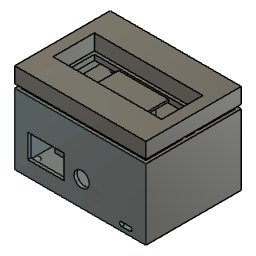
Todas la partes de la carcasa v1 (Autodesk Fusion 360 design; units mm, degrees)
Autodesk Fusion 360 part; units mm, degrees
(part 1 of 4)
sketch "Boceto1" plane through (0, 0, 0) normal (0, 1, 0) x (1, 0, 0)
sketch "Boceto2" plane through (0, 0, 0) normal (0, 1, 0) x (1, 0, 0)
  line L0 (-80, 70) -> (41, 70)
  line L1 (41, 70) -> (41, -16.3)
  line L2 (41, -16.3) -> (-80, -16.3)
  line L3 (-80, -16.3) -> (-80, 70)
  line L4 (44, -19.3) -> (-83, -19.3)
  line L5 (-83, -19.3) -> (-83, 73)
  line L6 (-83, 73) -> (44, 73)
  line L7 (44, 73) -> (44, -19.3)
  dimension "d1" = 121
  dimension "d2" = 86.3
  dimension "d3" = -3
  constraint horizontal L0
  constraint vertical L1
  constraint horizontal L2
  constraint vertical L3
  measures "d1" distance of L0.start L0.end
  measures "d2" distance of L0.end L1.end
extrude "Extruir1" add sketch "Boceto2" along normal blind 64.2 makes body 1
sketch "Boceto3" plane through (0, 0, 0) normal (0, 1, 0) x (1, 0, 0)
  line L0 (41, 70) -> (41, -16.3)
  line L1 (44, -19.3) -> (44, 73)
extrude "Extruir3" add sketch "Boceto2" against normal blind 4 contours L0 L1 L2 L3 | L4 L5 L6 L7 bodies 1
sketch "Boceto4" plane through (0, 0, 0) normal (0, 1, 0) x (1, 0, 0)
  line L0 (-47.2876, 12.1063) -> (-72.5876, 12.1063)
  line L1 (-45.7876, 61.8063) -> (-45.7876, 13.6063)
  circle A0 centre (-48.1876, 61.0063) radius 1.45
  circle A1 centre (-48.1876, 14.4063) radius 1.45
  line L2 (-72.5876, 12.1063) -> (-74.0876, 13.6063)
  line L3 (-47.2876, 12.1063) -> (-45.7876, 13.6063)
  circle A2 centre (-71.6876, 14.4063) radius 1.45
  line L4 (-45.7876, 13.6063) -> (-45.7876, 61.8063)
  line L5 (-45.7876, 61.8063) -> (-47.2876, 63.3063)
  circle A3 centre (-71.6876, 14.4063) radius 1.45
  line L6 (-72.5876, 63.3063) -> (-47.2876, 63.3063)
  line L7 (-74.0876, 13.6063) -> (-72.5876, 12.1063)
  line L8 (-74.0876, 61.8063) -> (-72.5876, 63.3063)
  circle A4 centre (-71.6876, 61.0063) radius 1.45
  line L9 (-72.5876, 12.1063) -> (-47.2876, 12.1063)
  line L10 (-72.5876, 63.3063) -> (-74.0876, 61.8063)
  line L11 (-74.0876, 61.8063) -> (-74.0876, 13.6063)
  circle A5 centre (-71.6876, 61.0063) radius 1.45
  line L12 (-74.0876, 13.6063) -> (-74.0876, 61.8063)
  circle A6 centre (-48.1876, 61.0063) radius 1.45
  line L13 (-47.2876, 63.3063) -> (-72.5876, 63.3063)
  line L14 (-45.7876, 13.6063) -> (-47.2876, 12.1063)
  line L15 (-47.2876, 63.3063) -> (-45.7876, 61.8063)
  circle A7 centre (-48.1876, 14.4063) radius 1.45
  line L16 (-43.7876, 12.7779) -> (-46.4591, 10.1063)
  line L17 (-73.416, 10.1063) -> (-46.4591, 10.1063)
  line L18 (-73.416, 10.1063) -> (-76.0876, 12.7779)
  line L19 (-76.0876, 62.6347) -> (-76.0876, 12.7779)
  line L20 (-76.0876, 62.6347) -> (-73.416, 65.3063)
  line L21 (-46.4591, 65.3063) -> (-73.416, 65.3063)
  line L22 (-46.4591, 65.3063) -> (-43.7876, 62.6347)
  line L23 (-43.7876, 62.6347) -> (-43.7876, 12.7779)
  point P0 (-45.7876, 63.3063)
  dimension "d10" = -2
sketch "Boceto5" plane through (0, 0, 0) normal (0, 1, 0) x (1, 0, 0)
extrude "Extruir4" add sketch "Boceto4" along normal blind 11 contours L16 L17 L18 L19 L20 L21 L22 L23 bodies 1
extrude "Extruir5" add sketch "Boceto4" along normal blind 9.866 contours A0 A6 | A1 A7 | A2 A3 | A4 A5 bodies 1
sketch "Boceto6" plane through (0, 0, 19.3) normal (0, 0, 1) x (1, 0, 0)
  line L0 (-70.6711, 11.1811) -> (-35.0211, 11.1811)
  line L1 (-35.0211, 34.2811) -> (-46.6399, 34.2811)
  circle A0 centre (-37.6711, 8.3311) radius 1.45
  line L2 (-35.0211, 39.3811) -> (-35.0211, 30.3811)
  line L3 (-45.8461, 39.3811) -> (-35.0211, 39.3811)
  line L4 (-70.6711, 34.2811) -> (-70.6711, 11.1811)
  line L5 (-35.0211, 5.7811) -> (-70.6711, 5.7811)
  line L6 (-35.0211, 11.1811) -> (-35.0211, 34.2811)
  line L7 (-59.0499, 34.2811) -> (-70.6711, 34.2811)
  line L8 (-46.6399, 34.2811) -> (-59.0499, 34.2811)
  circle A1 centre (-37.6711, 36.9311) radius 1.45
  line L9 (-35.0211, 11.1811) -> (-35.0211, 5.7811)
  circle A2 centre (-37.6711, 36.8311) radius 1.45
  line L10 (-35.0211, 33.9811) -> (-35.0211, 10.8811)
  line L11 (-45.8461, 5.7811) -> (-45.8461, 9.5311)
  line L12 (-59.8461, 9.5311) -> (-59.8461, 5.7811)
  line L13 (-70.6711, 14.7811) -> (-70.6711, 5.7811)
  line L14 (-46.6399, 10.8811) -> (-59.0499, 10.8811)
  line L15 (-35.0211, 33.9811) -> (-35.0211, 39.3811)
  line L16 (-70.6711, 10.8811) -> (-70.6711, 33.9811)
  line L17 (-59.0499, 10.8811) -> (-70.6711, 10.8811)
  line L18 (-45.8461, 9.5311) -> (-59.8461, 9.5311)
  line L19 (-70.6711, 5.7811) -> (-59.8461, 5.7811)
  line L20 (-35.0211, 39.3811) -> (-70.6711, 39.3811)
  line L21 (-70.6711, 39.3811) -> (-70.6711, 33.9811)
  line L22 (-70.6711, 33.9811) -> (-35.0211, 33.9811)
  line L23 (-35.0211, 10.8811) -> (-46.6399, 10.8811)
  line L24 (-35.0211, 5.7811) -> (-35.0211, 14.7811)
  circle A3 centre (-37.6711, 8.2311) radius 1.45
  circle A4 centre (-68.0211, 8.2311) radius 1.45
  circle A5 centre (-68.0211, 36.8311) radius 1.45
  point P0 (-52.8461, 22.5811)
  point P1 (-52.8461, 22.5811)
sketch "Boceto7" plane through (0, 0, 0) normal (0, 1, 0) x (1, 0, 0)
  line L0 (-6.4734, 52.2282) -> (33.9266, 52.2282)
  line L1 (-6.4738, 51.7714) -> (-6.4738, 57.7714)
  arc A0 (33.9266, 52.2282) -> (33.9266, 57.2282) centre (33.9266, 54.7282) ccw
  line L2 (-16.6738, 51.7714) -> (-6.4738, 51.7714)
  line L3 (-16.6738, 57.7714) -> (-16.6738, 51.7714)
  line L4 (33.9266, 57.2282) -> (-6.4734, 57.2282)
  line L5 (-6.4738, 57.7714) -> (-16.6738, 57.7714)
  point P0 (11.2266, 57.2282)
sketch "Boceto8" plane through (0, 0, 0) normal (0, 1, 0) x (1, 0, 0)
  line L0 (-6.2702, 42.1492) -> (34.1298, 42.1492)
  line L1 (-6.2705, 41.6923) -> (-6.2705, 47.6923)
  arc A0 (34.1298, 42.1492) -> (34.1298, 47.1492) centre (34.1298, 44.6492) ccw
  line L2 (-16.4705, 41.6923) -> (-6.2705, 41.6923)
  line L3 (-16.4705, 47.6923) -> (-16.4705, 41.6923)
  line L4 (34.1298, 47.1492) -> (-6.2702, 47.1492)
  line L5 (-6.2705, 47.6923) -> (-16.4705, 47.6923)
  point P0 (11.4298, 47.1492)
sketch "Boceto9" plane through (0, 0, 0) normal (0, 1, 0) x (1, 0, 0)
  line L0 (-6.3461, 32.1874) -> (34.0539, 32.1874)
  line L1 (-6.3465, 31.7305) -> (-6.3465, 37.7305)
  arc A0 (34.0539, 32.1874) -> (34.0539, 37.1874) centre (34.0539, 34.6874) ccw
  line L2 (-16.5465, 31.7305) -> (-6.3465, 31.7305)
  line L3 (-16.5465, 37.7305) -> (-16.5465, 31.7305)
  line L4 (34.0539, 37.1874) -> (-6.3461, 37.1874)
  line L5 (-6.3465, 37.7305) -> (-16.5465, 37.7305)
  point P0 (11.3539, 37.1874)
sketch "Boceto10" plane through (0, 0, 0) normal (0, 1, 0) x (-1, 0, 0)
  line L0 (-41, 16.3) -> (-41, -70)
  line L1 (-41, -70) -> (80, -70)
  line L2 (80, -70) -> (80, 16.3)
  line L3 (80, 16.3) -> (-41, 16.3)
  line L4 (46.4591, -65.3063) -> (43.7876, -62.6347)
  line L5 (43.7876, -62.6347) -> (43.7876, -12.7779)
  line L6 (43.7876, -12.7779) -> (46.4591, -10.1063)
  line L7 (46.4591, -10.1063) -> (73.416, -10.1063)
  line L8 (73.416, -10.1063) -> (76.0876, -12.7779)
  line L9 (76.0876, -12.7779) -> (76.0876, -62.6347)
  line L10 (76.0876, -62.6347) -> (73.416, -65.3063)
  line L11 (73.416, -65.3063) -> (46.4591, -65.3063)
  line L12 (6.3465, -31.7305) -> (6.3465, -37.7305)
  line L13 (16.5465, -31.7305) -> (6.3465, -31.7305)
  line L14 (6.3465, -37.7305) -> (16.5465, -37.7305)
  line L15 (16.5465, -37.7305) -> (16.5465, -31.7305)
  line L16 (-34.0539, -37.1874) -> (6.3461, -37.1874)
  line L17 (6.3461, -32.1874) -> (-34.0539, -32.1874)
  arc A0 (-34.0539, -32.1874) -> (-34.0539, -37.1874) centre (-34.0539, -34.6874) ccw
  line L18 (6.2702, -42.1492) -> (-34.1298, -42.1492)
  arc A1 (-34.1298, -42.1492) -> (-34.1298, -47.1492) centre (-34.1298, -44.6492) ccw
  line L19 (-34.1298, -47.1492) -> (6.2702, -47.1492)
  line L20 (16.4705, -47.6923) -> (16.4705, -41.6923)
  line L21 (16.4705, -41.6923) -> (6.2705, -41.6923)
  line L22 (6.2705, -41.6923) -> (6.2705, -47.6923)
  line L23 (6.2705, -47.6923) -> (16.4705, -47.6923)
  line L24 (6.4734, -52.2282) -> (-33.9266, -52.2282)
  arc A2 (-33.9266, -52.2282) -> (-33.9266, -57.2282) centre (-33.9266, -54.7282) ccw
  line L25 (-33.9266, -57.2282) -> (6.4734, -57.2282)
  line L26 (6.4738, -57.7714) -> (16.6738, -57.7714)
  line L27 (6.4738, -51.7714) -> (6.4738, -57.7714)
  line L28 (16.6738, -57.7714) -> (16.6738, -51.7714)
  line L29 (16.6738, -51.7714) -> (6.4738, -51.7714)
  line L30 (-38.4075, -28.7305) -> (19.6738, -28.7305)
  line L31 (19.6738, -28.7305) -> (19.6738, -60.7714)
  line L32 (19.6738, -60.7714) -> (-38.4075, -60.7714)
  line L33 (-38.4075, -60.7714) -> (-38.4075, -28.7305)
  line L34 (16.6738, -57.7714) -> (19.6738, -57.7714) construction
  line L35 (16.6738, -57.7714) -> (16.6738, -60.7714) construction
  line L36 (16.5465, -31.7305) -> (16.5091, -28.7305) construction
  line L37 (-36.6075, -44.9828) -> (-38.4075, -44.9828) construction
  dimension "d19" = 3
  dimension "d20" = 3
  dimension "d21" = 3
  dimension "d22" = 1.8
  constraint horizontal L30
  constraint vertical L31
  constraint horizontal L32
  constraint vertical L33
  constraint coincident L26.end L28.start
  constraint coincident L31 L34.end
  constraint perpendicular L31 L34
  constraint coincident L32 L35.end
  constraint perpendicular L32 L35
  constraint coincident L13.start L15.end
  constraint coincident L30 L36.end
  constraint coincident A1 L37.start
  constraint coincident L33 L37.end
  constraint perpendicular L33 L37
  measures "d19" distance of L26.end L34.end
  measures "d20" distance of L26.end L35.end
  measures "d21" vertical distance of L13.start L36.end
  measures "d22" distance of L37.start L37.end
extrude "Extruir8" add sketch "Boceto10" along normal blind 15 contours L12 L16 L17 A0 | L18 A1 L19 L22 | L24 A2 L25 L27 | L30 L31 L32 L33 bodies 1
sketch "Boceto11" plane through (0, 0, 0) normal (0, 1, 0) x (1, 0, 0)
sketch "Boceto12" plane through (0, 15, 0) normal (0, 1, 0) x (-1, 0, 0)
  line L0 (6.4738, -51.7714) -> (16.6738, -51.7714)
  line L1 (16.6738, -51.7714) -> (16.6738, -57.7714)
  line L2 (16.6738, -57.7714) -> (6.4738, -57.7714)
  line L3 (6.4738, -57.7714) -> (6.4738, -51.7714)
  line L4 (16.5465, -31.7305) -> (16.5465, -37.7305)
  line L5 (16.5465, -37.7305) -> (6.3465, -37.7305)
  line L6 (6.3465, -37.7305) -> (6.3465, -31.7305)
  line L7 (6.3465, -31.7305) -> (16.5465, -31.7305)
  line L8 (16.4705, -47.6923) -> (6.2705, -47.6923)
  line L9 (6.2705, -47.6923) -> (6.2705, -41.6923)
  line L10 (6.2705, -41.6923) -> (16.4705, -41.6923)
  line L11 (16.4705, -41.6923) -> (16.4705, -47.6923)
  line L12 (-38.4075, -60.7714) -> (19.6738, -60.7714)
  line L13 (19.6738, -60.7714) -> (19.6738, -28.7305)
  line L14 (19.6738, -28.7305) -> (-38.4075, -28.7305)
  line L15 (-38.4075, -28.7305) -> (-38.4075, -60.7714)
  line L16 (-33.9266, -57.2282) -> (6.4734, -57.2282)
  arc A0 (-33.9266, -52.2282) -> (-33.9266, -57.2282) centre (-33.9266, -54.7282) ccw
  line L17 (6.4734, -52.2282) -> (-33.9266, -52.2282)
  line L18 (6.4734, -57.2282) -> (-33.9266, -57.2282)
  line L19 (-33.9266, -57.2282) -> (-33.9266, -52.2282)
  line L20 (-33.9266, -52.2282) -> (6.4734, -52.2282)
  line L21 (6.4734, -52.2282) -> (6.4734, -57.2282)
  line L22 (-34.1298, -47.1492) -> (6.2702, -47.1492)
  line L23 (6.2702, -42.1492) -> (-34.1298, -42.1492)
  arc A1 (-34.1298, -42.1492) -> (-34.1298, -47.1492) centre (-34.1298, -44.6492) ccw
  line L24 (-34.0539, -37.1874) -> (6.3461, -37.1874)
  line L25 (6.3461, -32.1874) -> (-34.0539, -32.1874)
  arc A2 (-34.0539, -32.1874) -> (-34.0539, -37.1874) centre (-34.0539, -34.6874) ccw
  line L26 (6.2702, -47.1492) -> (-34.1298, -47.1492)
  line L27 (-34.1298, -47.1492) -> (-34.1298, -42.1492)
  line L28 (-34.1298, -42.1492) -> (6.2702, -42.1492)
  line L29 (6.2702, -42.1492) -> (6.2702, -47.1492)
  line L30 (6.3461, -37.1874) -> (-34.0539, -37.1874)
  line L31 (-34.0539, -37.1874) -> (-34.0539, -32.1874)
  line L32 (-34.0539, -32.1874) -> (6.3461, -32.1874)
  line L33 (6.3461, -32.1874) -> (6.3461, -37.1874)
  constraint horizontal L18
  constraint vertical L19
  constraint horizontal L20
  constraint vertical L21
  constraint coincident A0.start L17.end
  constraint coincident L16.end L18.start
  constraint horizontal L26
  constraint vertical L27
  constraint horizontal L28
  constraint vertical L29
  constraint coincident L23.end A1.start
  constraint coincident L22.end L26.start
  constraint horizontal L30
  constraint vertical L31
  constraint horizontal L32
  constraint vertical L33
  constraint coincident L25.end A2.start
  constraint coincident L24.end L30.start
extrude "Extruir9" cut sketch "Boceto12" against normal blind 15 contours L16 L17 L18 L19 L20 L21 | A0 L19 | L22 L23 L26 L27 L28 L29 | A1 L27 | L24 L25 L30 L31 L32 L33 | A2 L31 bodies 1
extrude "Extruir10" cut 1 faces at (-6.3461, 10, -33.854) along direction (-1, 0, 0) blind 3 on bodies 1 bodies 1
extrude "Extruir11" cut 1 faces at (-6.2702, 10, -43.8159) along direction (-1, 0, 0) blind 3 on bodies 1 bodies 1
extrude "Extruir12" cut 1 faces at (-6.4734, 10, -53.8949) along direction (-1, 0, 0) blind 2 on bodies 1 bodies 1
sketch "Boceto13" plane through (0, 0, 19.3) normal (0, 0, 1) x (1, 0, 0)
  circle A0 centre (-23.7062, 31.534) radius 1.5
  line L0 (-10.9162, 11.184) -> (-13.4262, 11.184)
  line L1 (-26.2062, 35.884) -> (-7.2062, 35.884)
  line L2 (-7.2062, 13.634) -> (-26.2062, 13.634)
  line L3 (-23.7062, 9.634) -> (-23.7062, 35.884)
  line L4 (-8.4062, 35.884) -> (-8.4062, 9.634)
  line L5 (-18.4462, 11.184) -> (-20.9562, 11.184)
  line L6 (-18.4462, 13.634) -> (-15.9362, 13.634)
  line L7 (-15.9362, 11.184) -> (-15.9362, 13.634)
  line L8 (-7.2062, 9.634) -> (-26.2062, 9.634)
  circle A1 centre (-23.7062, 14.684) radius 1.5
  line L9 (-20.9562, 35.884) -> (-20.9562, 9.634)
  line L10 (-20.9562, 13.634) -> (-18.4462, 13.634)
  line L11 (-26.2062, 31.534) -> (-7.2062, 31.534)
  line L12 (-7.2062, 9.634) -> (-26.2062, 35.884)
  line L13 (-26.2062, 9.634) -> (-26.2062, 35.884)
  line L14 (-26.2062, 9.634) -> (-7.2062, 35.884)
  line L15 (-23.7062, 31.534) -> (-23.7062, 14.684)
  line L16 (-18.4462, 13.634) -> (-18.4462, 11.184)
  line L17 (-7.2062, 11.184) -> (-26.2062, 11.184)
  line L18 (-20.9562, 11.184) -> (-20.9562, 13.634)
  line L19 (-15.9362, 13.634) -> (-15.9362, 11.184)
  line L20 (-15.9362, 11.184) -> (-18.4462, 11.184)
  line L21 (-18.4462, 11.184) -> (-18.4462, 13.634)
  line L22 (-13.4262, 13.634) -> (-13.4262, 11.184)
  line L23 (-13.4262, 11.184) -> (-15.9362, 11.184)
  line L24 (-13.4262, 13.634) -> (-10.9162, 13.634)
  line L25 (-10.9162, 13.634) -> (-10.9162, 11.184)
  line L26 (-13.4262, 11.184) -> (-13.4262, 13.634)
  line L27 (-10.9162, 13.634) -> (-8.4062, 13.634)
  line L28 (-8.4062, 13.634) -> (-8.4062, 11.184)
  line L29 (-15.9362, 13.634) -> (-13.4262, 13.634)
  line L30 (-7.2062, 35.884) -> (-7.2062, 9.634)
  line L31 (-18.4462, 12.409) -> (-15.9362, 12.409)
  line L32 (-15.9362, 12.409) -> (-13.4262, 12.409)
  line L33 (-10.9162, 11.184) -> (-10.9162, 13.634)
  line L34 (-8.4062, 11.184) -> (-10.9162, 11.184)
  circle A2 centre (-12.1712, 12.409) radius 0.5
  circle A3 centre (-17.1912, 12.409) radius 0.5
  line L35 (-13.4262, 12.409) -> (-10.9162, 12.409)
  circle A4 centre (-19.7012, 12.409) radius 0.5
  line L36 (-20.9562, 12.409) -> (-18.4462, 12.409)
  circle A5 centre (-9.6612, 12.409) radius 0.5
  line L37 (-10.9162, 12.409) -> (-8.4062, 12.409)
  circle A6 centre (-14.6812, 12.409) radius 0.5
  line L38 (-11.1762, 19.324) -> (-12.6762, 19.324)
  line L39 (-14.4062, 31.224) -> (-15.9062, 32.874)
  line L40 (-21.1062, 19.324) -> (-9.2062, 19.324)
  line L41 (-18.3862, 31.224) -> (-18.3862, 32.874)
  line L42 (-7.2062, 35.884) -> (-7.2062, 9.634)
  line L43 (-11.9262, 25.274) -> (-11.9262, 31.224)
  line L44 (-15.9062, 32.874) -> (-14.4062, 32.874)
  line L45 (-14.4062, 31.224) -> (-15.9062, 31.224)
  line L46 (-15.1562, 31.224) -> (-15.1562, 32.874)
  line L47 (-15.9062, 31.224) -> (-14.4062, 32.874)
  line L48 (-11.1762, 31.224) -> (-12.6762, 31.224)
  line L49 (-19.1362, 31.224) -> (-19.1362, 32.874)
  line L50 (-12.6762, 32.874) -> (-11.1762, 32.874)
  line L51 (-19.1362, 32.874) -> (-17.6362, 32.874)
  line L52 (-9.2062, 35.884) -> (-9.2062, 9.634)
  line L53 (-17.6362, 32.874) -> (-17.6362, 31.224)
  line L54 (-19.1362, 31.224) -> (-17.6362, 32.874)
  line L55 (-21.1062, 31.224) -> (-21.1062, 19.324)
  line L56 (-9.2062, 19.324) -> (-9.2062, 31.224)
  line L57 (-11.9262, 19.324) -> (-11.9262, 18.224)
  line L58 (-11.1762, 19.324) -> (-12.6762, 18.224)
  line L59 (-12.6762, 19.324) -> (-11.1762, 18.224)
  line L60 (-12.6762, 19.324) -> (-12.6762, 18.224)
  line L61 (-11.1762, 18.224) -> (-11.1762, 19.324)
  line L62 (-17.6362, 31.224) -> (-19.1362, 32.874)
  line L63 (-9.2062, 31.224) -> (-21.1062, 31.224)
  line L64 (-12.6762, 18.224) -> (-11.1762, 18.224)
  line L65 (-18.3862, 19.324) -> (-18.3862, 18.224)
  line L66 (-15.9062, 31.224) -> (-15.9062, 32.874)
  line L67 (-11.1762, 31.224) -> (-12.6762, 32.874)
  line L68 (-12.6762, 31.224) -> (-11.1762, 32.874)
  line L69 (-14.4062, 32.874) -> (-14.4062, 31.224)
  line L70 (-17.6362, 31.224) -> (-19.1362, 31.224)
  line L71 (-26.2062, 35.884) -> (-7.2062, 35.884)
  line L72 (-17.6362, 19.324) -> (-19.1362, 19.324)
  line L73 (-19.1362, 19.324) -> (-19.1362, 18.224)
  line L74 (-18.3862, 25.274) -> (-18.3862, 19.324)
  line L75 (-18.3862, 25.274) -> (-18.3862, 31.224)
  line L76 (-11.1762, 32.874) -> (-11.1762, 31.224)
  line L77 (-19.1362, 18.224) -> (-17.6362, 18.224)
  line L78 (-11.9262, 31.224) -> (-11.9262, 32.874)
  line L79 (-17.6362, 18.224) -> (-17.6362, 19.324)
  line L80 (-26.2062, 31.224) -> (-7.2062, 31.224)
  line L81 (-15.1562, 31.224) -> (-15.1562, 19.324)
  line L82 (-18.3862, 25.274) -> (-11.9262, 25.274)
  line L83 (-11.9262, 25.274) -> (-11.9262, 19.324)
  line L84 (-12.6762, 31.224) -> (-12.6762, 32.874)
  circle A7 centre (-18.3862, 32.874) radius 0.5
  line L85 (-17.6362, 19.324) -> (-19.1362, 18.224)
  circle A8 centre (-11.9262, 18.224) radius 0.5
  line L86 (-19.1362, 19.324) -> (-17.6362, 18.224)
  circle A9 centre (-18.3862, 18.224) radius 0.5
  circle A10 centre (-15.1562, 32.874) radius 0.5
  circle A11 centre (-11.9262, 32.874) radius 0.5
  line L87 (-6.7412, 22.759) -> (-6.7412, 24.259)
  line L88 (-20.1412, 24.109) -> (-21.2412, 24.109)
  line L89 (-21.0912, 24.259) -> (-21.0912, 22.759)
  line L90 (-8.2412, 24.259) -> (-8.2412, 22.759)
  line L91 (-6.5912, 24.109) -> (-8.2412, 24.109)
  line L92 (-21.2412, 22.759) -> (-20.1412, 22.759)
  line L93 (-21.2412, 24.259) -> (-21.2412, 22.759)
  line L94 (-20.1412, 22.759) -> (-20.1412, 24.259)
  line L95 (-6.5912, 22.759) -> (-6.5912, 24.259)
  line L96 (-6.5912, 24.259) -> (-8.2412, 24.259)
  line L97 (-8.2412, 22.759) -> (-6.5912, 22.759)
  line L98 (-20.1412, 24.259) -> (-21.2412, 24.259)
  line L99 (-23.4262, 33.434) -> (-23.4262, 32.784)
  line L100 (-12.4562, 33.109) -> (-14.9662, 33.109)
  line L101 (-24.0762, 32.784) -> (-24.0762, 33.434)
  line L102 (-15.8962, 33.434) -> (-16.5462, 32.784)
  line L103 (-21.5662, 32.784) -> (-21.5662, 33.434)
  line L104 (-14.0362, 33.434) -> (-13.3862, 32.784)
  line L105 (-13.3862, 33.434) -> (-14.0362, 32.784)
  line L106 (-19.0562, 32.784) -> (-19.0562, 33.434)
  line L107 (-20.9162, 32.784) -> (-21.5662, 32.784)
  line L108 (-24.0762, 33.434) -> (-23.4262, 33.434)
  line L109 (-23.4262, 32.784) -> (-24.0762, 32.784)
  line L110 (-15.8962, 33.434) -> (-15.8962, 32.784)
  line L111 (-13.3862, 32.784) -> (-14.0362, 32.784)
  line L112 (-14.0362, 32.784) -> (-14.0362, 33.434)
  line L113 (-19.9862, 33.109) -> (-22.4962, 33.109)
  line L114 (-22.4962, 33.109) -> (-25.0062, 33.109)
  line L115 (-16.5462, 33.434) -> (-15.8962, 32.784)
  line L116 (-16.5462, 32.784) -> (-16.5462, 33.434)
  line L117 (-19.0562, 33.434) -> (-18.4062, 33.434)
  line L118 (-21.5662, 33.434) -> (-20.9162, 32.784)
  line L119 (-13.3862, 32.784) -> (-14.0362, 32.784)
  line L120 (-20.9162, 33.434) -> (-21.5662, 32.784)
  line L121 (-24.0762, 33.434) -> (-23.4262, 32.784)
  line L122 (-23.4262, 33.434) -> (-24.0762, 32.784)
  line L123 (-17.4762, 33.109) -> (-19.9862, 33.109)
  line L124 (-16.5462, 33.434) -> (-15.8962, 33.434)
  line L125 (-14.0362, 32.784) -> (-14.0362, 40.384)
  line L126 (-14.0362, 40.384) -> (-13.3862, 40.384)
  line L127 (-14.9662, 33.109) -> (-17.4762, 33.109)
  line L128 (-19.0562, 33.434) -> (-18.4062, 32.784)
  line L129 (-21.5662, 33.434) -> (-20.9162, 33.434)
  line L130 (-20.9162, 33.434) -> (-20.9162, 32.784)
  line L131 (-14.0362, 33.434) -> (-13.3862, 33.434)
  line L132 (-18.4062, 32.784) -> (-19.0562, 32.784)
  line L133 (-15.8962, 32.784) -> (-16.5462, 32.784)
  line L134 (-18.4062, 33.434) -> (-18.4062, 32.784)
  line L135 (-18.4062, 33.434) -> (-19.0562, 32.784)
  line L136 (-13.3862, 33.434) -> (-13.3862, 32.784)
  line L137 (-15.8962, 32.784) -> (-16.5462, 32.784)
  line L138 (-15.8962, 40.384) -> (-15.8962, 32.784)
  line L139 (-16.5462, 32.784) -> (-16.5462, 40.384)
  line L140 (-18.4062, 40.384) -> (-18.4062, 32.784)
  line L141 (-23.4262, 32.784) -> (-24.0762, 32.784)
  line L142 (-18.4062, 32.784) -> (-19.0562, 32.784)
  line L143 (-19.0562, 32.784) -> (-19.0562, 40.384)
  line L144 (-23.4262, 40.384) -> (-23.4262, 32.784)
  line L145 (-20.9162, 40.384) -> (-20.9162, 32.784)
  line L146 (-21.5662, 32.784) -> (-21.5662, 40.384)
  line L147 (-19.0562, 40.384) -> (-18.4062, 40.384)
  line L148 (-21.5662, 40.384) -> (-20.9162, 40.384)
  line L149 (-24.0762, 40.384) -> (-23.4262, 40.384)
  line L150 (-16.5462, 40.384) -> (-15.8962, 40.384)
  line L151 (-13.3862, 40.384) -> (-13.3862, 32.784)
  line L152 (-24.0762, 32.784) -> (-24.0762, 40.384)
  line L153 (-20.9162, 32.784) -> (-21.5662, 32.784)
  line L154 (-27.3812, 25.359) -> (-27.3812, 27.209)
  line L155 (-34.3312, 25.359) -> (-26.7312, 25.359)
  line L156 (-34.3312, 27.209) -> (-34.3312, 25.359)
  line L157 (-26.7312, 27.209) -> (-34.3312, 27.209)
  line L158 (-26.7312, 26.559) -> (-34.3312, 26.559)
  line L159 (-26.7312, 25.359) -> (-26.7312, 27.209)
  line L160 (-12.3062, 20.244) -> (-24.2062, 20.244)
  circle A12 centre (-18.2562, 20.244) radius 2
  circle A13 centre (-18.2562, 20.244) radius 3.5
  line L161 (-24.2062, 25.944) -> (-24.2062, 14.544)
  line L162 (-12.5562, 14.294) -> (-12.3062, 14.544)
  line L163 (-12.3062, 14.544) -> (-12.3062, 25.944)
  line L164 (-23.9562, 26.194) -> (-24.2062, 25.944)
  line L165 (-12.3062, 25.944) -> (-12.5562, 26.194)
  line L166 (-24.2062, 14.544) -> (-23.9562, 14.294)
  line L167 (-23.9562, 14.294) -> (-12.5562, 14.294)
  line L168 (-12.5562, 26.194) -> (-23.9562, 26.194)
  circle A14 centre (-18.2562, 20.244) radius 3
  circle A15 centre (-18.2562, 20.244) radius 2
  line L169 (-15.6581, 21.744) -> (-20.8543, 21.744)
  line L170 (-18.2562, 17.244) -> (-18.2562, 21.744)
  circle A16 centre (-18.2562, 20.244) radius 3
  circle A17 centre (-16.7062, 25.009) radius 3
  circle A18 centre (-16.7062, 25.009) radius 6.49
  circle A19 centre (-16.7062, 25.009) radius 7.04
  circle A20 centre (-18.2562, 20.244) radius 6.49
  circle A21 centre (-18.2562, 20.244) radius 7.04
  circle A22 centre (-18.2562, 20.244) radius 7.405
  circle A23 centre (-18.2562, 20.244) radius 7.04
  circle A24 centre (-18.2562, 20.244) radius 7.04
  line L171 (-25.6597, 20.094) -> (-25.4946, 20.094)
  circle A25 centre (-18.2562, 20.244) radius 7.405
  circle A26 centre (-18.2562, 20.244) radius 7.24
  line L172 (-11.0177, 20.394) -> (-10.8527, 20.394)
  line L173 (-11.0162, 20.244) -> (-10.8512, 20.244)
  line L174 (-11.0177, 20.094) -> (-10.8527, 20.094)
  line L175 (-25.6612, 20.244) -> (-25.4962, 20.244)
  circle A27 centre (-18.2562, 20.244) radius 7.04
  line L176 (-25.6597, 20.394) -> (-25.4946, 20.394)
  line L177 (-23.3756, 25.3635) -> (-23.3852, 25.5852)
  line L178 (-11.5673, 23.0147) -> (-11.4149, 23.0778)
  line L179 (-11.5113, 22.8755) -> (-11.3589, 22.9387)
  line L180 (-25.0387, 17.2723) -> (-24.8862, 17.3354)
  line L181 (-18.2562, 27.484) -> (-18.1062, 27.6475)
  line L182 (-15.5616, 13.3467) -> (-15.4856, 13.5552)
  line L183 (-15.4224, 13.4027) -> (-15.4856, 13.5552)
  line L184 (-24.9451, 17.4734) -> (-25.0387, 17.2723)
  line L185 (-25.1535, 17.5494) -> (-25.001, 17.6126)
  line L186 (-13.1272, 25.5852) -> (-13.1367, 25.3635)
  line L187 (-15.2844, 27.0266) -> (-15.4856, 26.9329)
  line L188 (-23.4923, 15.0079) -> (-23.3756, 15.1246)
  line L189 (-10.8527, 20.394) -> (-11.0162, 20.244)
  line L190 (-15.6247, 26.9889) -> (-15.5616, 27.1414)
  line L191 (-21.09, 13.4027) -> (-21.0268, 13.5552)
  line L192 (-18.4062, 12.8406) -> (-18.2562, 13.004)
  line L193 (-18.4062, 27.6475) -> (-18.2562, 27.484)
  line L194 (-15.5616, 13.3467) -> (-15.6247, 13.4992)
  line L195 (-15.4856, 13.5552) -> (-15.2844, 13.4615)
  line L196 (-11.4737, 23.2158) -> (-11.5673, 23.0147)
  line L197 (-11.5673, 23.0147) -> (-11.3589, 22.9387)
  line L198 (-15.4856, 26.9329) -> (-15.4224, 27.0854)
  line L199 (-20.9508, 13.3467) -> (-20.8876, 13.4992)
  line L200 (-23.3756, 15.1246) -> (-23.3852, 14.9029)
  line L201 (-21.228, 13.4615) -> (-21.1648, 13.614)
  line L202 (-21.228, 27.0266) -> (-21.0268, 26.9329)
  line L203 (-15.5616, 27.1414) -> (-15.4856, 26.9329)
  line L204 (-15.3476, 26.8741) -> (-15.2844, 27.0266)
  line L205 (-13.1272, 14.9029) -> (-13.2439, 15.0196)
  line L206 (-13.1272, 14.9029) -> (-13.1367, 15.1246)
  line L207 (-18.2562, 13.004) -> (-18.1062, 12.8406)
  line L208 (-23.5973, 15.1151) -> (-23.4806, 15.2318)
  line L209 (-13.1367, 25.3635) -> (-13.0201, 25.4802)
  line L210 (-21.0268, 13.5552) -> (-20.9508, 13.3467)
  line L211 (-25.1535, 17.5494) -> (-24.9451, 17.4734)
  line L212 (-13.0318, 25.2563) -> (-12.9151, 25.373)
  line L213 (-23.5973, 15.1151) -> (-23.3756, 15.1246)
  line L214 (-21.228, 13.4615) -> (-21.0268, 13.5552)
  line L215 (-18.1062, 27.4825) -> (-18.1062, 27.6475)
  line L216 (-18.4062, 27.4825) -> (-18.4062, 27.6475)
  line L217 (-11.0162, 20.244) -> (-10.8527, 20.094)
  line L218 (-13.1367, 25.3635) -> (-12.9151, 25.373)
  line L219 (-25.6597, 20.394) -> (-25.4962, 20.244)
  line L220 (-25.6597, 20.094) -> (-25.4962, 20.244)
  line L221 (-25.0975, 17.4103) -> (-24.9451, 17.4734)
  line L222 (-11.6261, 23.1527) -> (-11.4737, 23.2158)
  line L223 (-18.2562, 12.839) -> (-18.2562, 13.004)
  line L224 (-15.2844, 13.4615) -> (-15.3476, 13.614)
  line L225 (-21.1648, 26.8741) -> (-21.228, 27.0266)
  line L226 (-20.8876, 26.9889) -> (-20.9508, 27.1414)
  line L227 (-18.4062, 12.8406) -> (-18.4062, 13.0056)
  line L228 (-13.0201, 15.0079) -> (-13.1367, 15.1246)
  line L229 (-12.9151, 15.1151) -> (-13.0318, 15.2318)
  line L230 (-23.2685, 25.4685) -> (-23.3852, 25.5852)
  line L231 (-13.1367, 15.1246) -> (-12.9151, 15.1151)
  line L232 (-23.3756, 25.3635) -> (-23.4923, 25.4802)
  line L233 (-21.0268, 26.9329) -> (-21.09, 27.0854)
  line L234 (-21.0268, 26.9329) -> (-20.9508, 27.1414)
  line L235 (-18.1062, 12.8406) -> (-18.1062, 13.0056)
  line L236 (-23.5973, 25.373) -> (-23.3756, 25.3635)
  line L237 (-23.3852, 14.9029) -> (-23.2685, 15.0196)
  line L238 (-13.2439, 25.4685) -> (-13.1272, 25.5852)
  line L239 (-18.2562, 27.484) -> (-18.2562, 27.649)
  line L240 (-23.4806, 25.2563) -> (-23.5973, 25.373)
  line L241 (-24.9451, 23.0147) -> (-25.0975, 23.0778)
  line L242 (-25.001, 22.8755) -> (-25.1535, 22.9387)
  line L243 (-25.1535, 22.9387) -> (-24.9451, 23.0147)
  line L244 (-24.9451, 23.0147) -> (-25.0387, 23.2158)
  line L245 (-24.8862, 23.1527) -> (-25.0387, 23.2158)
  line L246 (-11.3589, 17.5494) -> (-11.5673, 17.4734)
  line L247 (-11.5673, 17.4734) -> (-11.4737, 17.2723)
  line L248 (-11.4737, 17.2723) -> (-11.6261, 17.3354)
  line L249 (-11.4149, 17.4103) -> (-11.5673, 17.4734)
  line L250 (-11.3589, 17.5494) -> (-11.5113, 17.6126)
  line L251 (-18.0562, 27.034) -> (-18.0562, 25.034)
  line L252 (-18.5062, 27.034) -> (-18.5062, 25.034)
  line L253 (-18.0562, 25.034) -> (-18.5062, 25.034)
  line L254 (-18.0562, 27.4696) -> (-18.0562, 27.034)
  line L255 (-18.5062, 27.034) -> (-18.5062, 27.4696)
  line L256 (-18.2562, 27.034) -> (-18.2562, 25.034)
  line L257 (-18.2562, 20.244) -> (-18.2562, 27.034)
  line L258 (-18.0562, 27.034) -> (-18.5062, 27.034)
  line L259 (-18.5062, 27.4696) -> (-18.0562, 27.4696)
  circle A28 centre (-18.2562, 20.244) radius 6.79
  line L260 (-7.2062, 31.534) -> (-26.2062, 31.534)
  circle A29 centre (-16.2212, 33.109) radius 0.5
  circle A30 centre (-21.2412, 33.109) radius 0.5
  line L261 (-15.7212, 31.534) -> (-15.7212, 28.5934)
  circle A31 centre (-13.7112, 33.109) radius 0.5
  line L262 (-7.2062, 9.634) -> (-7.2062, 35.884)
  line L263 (-18.2312, 31.534) -> (-18.2312, 28.5934)
  line L264 (-23.2512, 31.534) -> (-23.2512, 28.5934)
  line L265 (-20.7412, 31.534) -> (-20.7412, 28.5934)
  line L266 (-13.2112, 31.534) -> (-13.2112, 28.5934)
  circle A32 centre (-9.7062, 13.984) radius 1.5
  circle A33 centre (-21.4862, 27.294) radius 0.5
  line L267 (-26.2062, 9.634) -> (-7.2062, 9.634)
  circle A34 centre (-18.2562, 12.644) radius 0.5
  line L268 (-7.2062, 28.5934) -> (-26.2062, 28.5934)
  circle A35 centre (-23.7512, 33.109) radius 0.5
  circle A36 centre (-15.0262, 12.644) radius 0.5
  circle A37 centre (-18.7312, 33.109) radius 0.5
  line L269 (-26.2062, 35.884) -> (-26.2062, 9.634)
  line L270 (-7.2062, 35.884) -> (-26.2062, 35.884)
  circle A38 centre (-15.0262, 27.294) radius 0.5
  circle A39 centre (-21.4862, 12.644) radius 0.5
  circle A40 centre (-9.7062, 30.834) radius 1.5
  circle A41 centre (-23.7062, 14.684) radius 1.5
  line L271 (-26.2062, 9.634) -> (-7.2062, 9.634)
  line L272 (-26.2062, 35.884) -> (-26.2062, 9.634)
  circle A42 centre (-23.7062, 31.534) radius 1.5
  line L273 (-7.2062, 9.634) -> (-7.2062, 35.884)
  circle A43 centre (-15.1562, 25.274) radius 7.04
  line L274 (-7.2062, 35.884) -> (-26.2062, 35.884)
  circle A44 centre (-16.7062, 25.009) radius 7.04
  circle A45 centre (-16.7062, 25.009) radius 7.04
  point P0 (-16.7062, 22.759)
  point P1 (-16.7062, 22.759)
  point P2 (-16.7062, 22.759)
  point P3 (-11.9262, 32.049)
  point P4 (-18.3862, 32.049)
  point P5 (-18.3862, 18.774)
  point P6 (-15.1562, 32.049)
  point P7 (-11.9262, 18.774)
  point P8 (-16.7062, 22.759)
  point P9 (-16.7062, 22.759)
  point P10 (-18.7312, 33.109)
  point P11 (-13.7112, 33.109)
  point P12 (-21.2412, 33.109)
  point P13 (-23.7512, 33.109)
  point P14 (-16.2212, 33.109)
  point P15 (-16.7062, 22.759)
  point P16 (-16.7062, 22.759)
  point P17 (-16.7062, 22.759)
  point P18 (-16.7062, 22.759)
  point P19 (-16.7062, 22.759)
  point P20 (-16.7062, 22.759)
  point P21 (-16.7062, 22.759)
  point P22 (-16.7062, 22.759)
  point P23 (-16.7062, 22.759)
  point P24 (-16.7062, 22.759)
  point P25 (-16.7062, 22.759)
  dimension "d35" = 14.08
  constraint concentric A19 A44
  constraint concentric A44 A45
  measures "d35" diameter of A45
extrude "Extruir14" add sketch "Boceto13" against normal blind 11.79 contours L11 L14 L52 L260 A40 | L11 L14 L260 A40 | L4 L11 L52 L260 A40 | L4 L11 L260 A40 | L11 L14 L63 L80 L260 A40 | L11 L14 L52 L63 L80 L260 | L4 L11 L52 L80 L260 | L2 L24 L25 L33 A32 | L2 L12 L25 L27 L33 A5 A32 | L12 A5 A32 | L4 L11 L80 L260 A40 | L14 L52 L56 L63 L80 A40 A43 | L14 L63 L80 A40 A43 | L4 L52 L56 L80 A40 | L2 L4 L27 L28 A5 L52 A32 | L2 L4 L28 A32 | L2 L4 A32 | L2 L12 L24 L27 A32 | L12 A5 L52 A32 | L2 L12 L27 A5 L52 | A5 L52 A32 | L4 L80 A40 | L14 A40 A43 | L14 A40 A43 | L2 L4 L27 L52 A32 | L2 L12 L27 L52 A32 bodies 1
sketch "Boceto14" plane through (0, 0, 19.3) normal (0, 0, 1) x (1, 0, 0)
  line L0 (44, -4) -> (44, 64.2)
  line L1 (44, 64.2) -> (-83, 64.2)
  line L2 (-83, 64.2) -> (-83, -4)
  line L3 (-83, -4) -> (44, -4)
  circle A0 centre (-18.2562, 20.244) radius 7.405
extrude "Extruir15" cut sketch "Boceto14" against normal blind 10 contours A0 bodies 1
sketch "Boceto18" plane through (44, 0, 0) normal (1, 0, 0) x (0, 0, -1)
  circle A0 centre (6.8601, 2.6386) radius 0.55
  line L0 (10.1484, -7.5902) -> (9.3984, -7.5902)
  line L1 (10.1484, -9.7902) -> (10.1484, -7.5902)
  line L2 (9.3984, 5.2098) -> (10.1484, 5.2098)
  line L3 (10.1484, 5.2098) -> (10.1484, 7.4098)
  circle A1 centre (6.8599, -4.6344) radius 0.55
  circle A2 centre (-15.6515, 5.8759) radius 0.55
  line L4 (-17.3516, 7.4098) -> (-17.3516, -9.7902)
  arc A3 (9.3984, 5.2098) -> (8.5484, 4.3598) centre (9.3984, 4.3598) ccw
  circle A4 centre (-15.6515, -8.2563) radius 0.55
  line L5 (-17.3516, -9.7902) -> (10.1484, -9.7902)
  line L6 (10.1484, 7.4098) -> (-17.3516, 7.4098)
  arc A5 (8.5484, -6.7402) -> (9.3984, -7.5902) centre (9.3984, -6.7402) ccw
  line L7 (8.5484, -6.7402) -> (8.5484, 4.3598)
  circle A6 centre (6.86, 5.8759) radius 0.55
  circle A7 centre (6.86, -8.2563) radius 0.55
  ellipse E0 centre (-7.6018, 1.9276) end of major axis (-7.6018, 2.1276) minor radius 0.1744 (-7.6018, 2.1276) -> (-7.7099, 2.0846) ccw
  line L8 (-7.6018, 2.1276) -> (-7.4407, 2.1276)
  arc A8 (-6.9349, 2.7526) -> (-7.4349, 2.2526) centre (-6.9349, 2.2526) ccw
  line L9 (-7.7099, 2.0846) -> (-7.7099, 1.9276)
  line L10 (-7.4349, 2.2526) -> (-7.4349, 2.1276)
  line L11 (-7.1349, 2.1276) -> (-7.1349, 2.2526)
  line L12 (-6.9349, 2.4526) -> (-6.7849, 2.4526)
  line L13 (-6.7849, 2.4526) -> (-6.7849, 2.7526)
  arc A9 (-6.9349, 2.4526) -> (-7.1349, 2.2526) centre (-6.9349, 2.2526) ccw
  line L14 (-6.7849, 2.7526) -> (-6.9349, 2.7526)
  line L15 (-7.4349, 2.1276) -> (-7.1349, 2.1276)
  arc A10 (-6.9349, 2.7526) -> (-7.4349, 2.2526) centre (-6.9349, 2.2526) ccw
  line L16 (-7.4349, 2.2526) -> (-7.4349, 2.1276)
  line L17 (-3.8949, 0.0276) -> (-3.738, 0.0276)
  line L18 (-6.7849, 2.9195) -> (-6.7849, 2.7584)
  arc A11 (-6.6556, 0.4491) -> (-6.3021, 0.3026) centre (-6.3021, 0.8026) ccw
  arc A12 (0.0651, 2.2526) -> (-0.4349, 2.7526) centre (-0.4349, 2.2526) ccw
  line L19 (-6.7849, 2.7526) -> (-6.9349, 2.7526)
  line L20 (0.3401, 1.9276) -> (0.3401, 1.8276)
  line L21 (0.0651, 2.1276) -> (0.0651, 2.2526)
  ellipse E1 centre (-6.5849, 2.9195) end of major axis (-6.7849, 2.9195) minor radius 0.1744 (-6.7418, 3.0276) -> (-6.7849, 2.9195) ccw
  line L22 (-7.7099, 1.9276) -> (-7.7099, 1.8276)
  line L23 (-3.6418, 0.0276) -> (-3.4849, 0.0276)
  line L24 (0.0709, 1.6276) -> (0.232, 1.6276)
  line L25 (-0.7142, 0.4491) -> (-0.0813, 1.0819)
  arc A13 (-7.4349, 1.4355) -> (-7.2885, 1.0819) centre (-6.9349, 1.4355) ccw
  line L26 (-6.2418, 0.0276) -> (-6.0849, 0.0276)
  line L27 (0.0651, 1.4355) -> (0.0651, 1.6276)
  ellipse E2 centre (0.232, 1.8276) end of major axis (0.232, 2.0276) minor radius 0.1744 (0.232, 1.6276) -> (0.3401, 1.6707) ccw
  line L28 (-7.7099, 1.8276) -> (-7.7099, 1.6707)
  ellipse E3 centre (-7.6018, 1.8276) end of major axis (-7.6018, 1.6276) minor radius 0.1744 (-7.7099, 1.6707) -> (-7.6018, 1.6276) ccw
  line L29 (-6.3021, 0.3026) -> (-6.2849, 0.3026)
  line L30 (-6.2849, 0.3526) -> (-6.2849, 0.2968)
  line L31 (0.3401, 1.6707) -> (0.3401, 1.8276)
  arc A14 (-0.0813, 1.0819) -> (0.0651, 1.4355) centre (-0.4349, 1.4355) ccw
  ellipse E4 centre (-6.0849, 0.1357) end of major axis (-5.8849, 0.1357) minor radius 0.1744 (-6.2849, 0.1357) -> (-6.2418, 0.0276) ccw
  ellipse E5 centre (-1.2849, 0.1357) end of major axis (-1.4849, 0.1357) minor radius 0.1744 (-1.128, 0.0276) -> (-1.0849, 0.1357) ccw
  line L32 (0.3401, 1.9276) -> (0.3401, 2.0846)
  line L33 (-0.7849, 3.0276) -> (-6.5849, 3.0276)
  line L34 (-6.5849, 3.0276) -> (-6.7418, 3.0276)
  ellipse E6 centre (0.232, 1.9276) end of major axis (0.232, 1.7276) minor radius 0.1744 (0.3401, 2.0846) -> (0.232, 2.1276) ccw
  line L35 (-0.5849, 2.9195) -> (-0.5849, 2.7584)
  line L36 (-7.4349, 1.6276) -> (-7.4349, 1.4355)
  line L37 (-1.2849, 0.0276) -> (-1.128, 0.0276)
  line L38 (-7.2885, 1.0819) -> (-6.6556, 0.4491)
  line L39 (-1.0849, 0.2968) -> (-1.0849, 0.1357)
  line L40 (0.0709, 2.1276) -> (0.232, 2.1276)
  ellipse E7 centre (-0.7849, 2.9195) end of major axis (-0.5849, 2.9195) minor radius 0.1744 (-0.5849, 2.9195) -> (-0.628, 3.0276) ccw
  line L41 (-6.2849, 0.2968) -> (-6.2849, 0.1357)
  line L42 (-1.2849, 0.0276) -> (-3.4849, 0.0276)
  line L43 (-7.6018, 1.6276) -> (-7.4407, 1.6276)
  line L44 (-0.4349, 2.7526) -> (-0.5849, 2.7526)
  line L45 (-3.8949, 0.0276) -> (-6.0849, 0.0276)
  arc A15 (-1.0677, 0.3026) -> (-0.7142, 0.4491) centre (-1.0677, 0.8026) ccw
  line L46 (-0.628, 3.0276) -> (-0.7849, 3.0276)
  point P0 (-3.6016, -1.1902)
  point P1 (-3.6016, -1.1902)
sketch "Boceto20" plane through (0, 0, 16.3) normal (0, 0, -1) x (-1, 0, 0)
  circle A0 centre (18.2562, 20.244) radius 7.405
  circle A1 centre (9.7062, 13.984) radius 1.5
  circle A2 centre (9.7062, 30.834) radius 1.5
  line L0 (-41, 0) -> (80, 0)
  line L1 (80, 0) -> (80, 64.2)
  line L2 (80, 64.2) -> (-41, 64.2)
  line L3 (-41, 64.2) -> (-41, 0)
  line L4 (80, 0) -> (80, 40)
  line L5 (80, 40) -> (74, 40)
  line L6 (74, 40) -> (74, 43)
  line L7 (74, 43) -> (80, 43)
  line L8 (80, 43) -> (80, 40)
  line L9 (-41, 0) -> (-41, 40)
  line L10 (-41, 40) -> (-35, 40)
  line L11 (-35, 40) -> (-35, 43)
  line L12 (-35, 43) -> (-41, 43)
  line L13 (-41, 43) -> (-41, 40)
  dimension "d64" = 40
  dimension "d65" = 3
  dimension "d66" = 6
  dimension "d67" = 3
  dimension "d68" = 6
  constraint coincident L0.end L1.start
  constraint perpendicular L0 L4
  constraint horizontal L5
  constraint vertical L6
  constraint horizontal L7
  constraint vertical L8
  constraint coincident L0.start L3.end
  constraint coincident L3 L9.end
  constraint horizontal L10
  constraint vertical L11
  constraint horizontal L12
  constraint vertical L13
  measures "d64" distance of L0.end L4.end
  measures "d65" distance of L4.end L7.end
  measures "d66" distance of L9.end L10.end
  measures "d67" distance of L9.end L12.end
  measures "d68" distance of L4.end L5.end
extrude "Extruir20" add sketch "Boceto20" along normal blind 86.3 contours L3 L10 L11 L12 L13 | L1 L5 L6 L7 L8 bodies 1
sketch "Boceto21" plane through (-80, 0, 0) normal (1, 0, 0) x (0, 0, -1)
  line L0 (-16.3, 43) -> (70, 43)
  line L1 (70, 43) -> (70, 64.2)
  line L2 (70, 64.2) -> (-16.3, 64.2)
  line L3 (-16.3, 64.2) -> (-16.3, 43)
  line L4 (-16.3, 43) -> (26.85, 43)
  line L5 (26.85, 43) -> (30.85, 43)
  line L6 (30.85, 43) -> (34.85, 43)
  line L7 (34.85, 43) -> (34.85, 64.2)
  line L8 (34.85, 64.2) -> (30.85, 64.2)
  line L9 (30.85, 64.2) -> (30.85, 43)
  line L10 (26.85, 43) -> (22.85, 43)
  line L11 (22.85, 43) -> (18.85, 43)
  line L12 (18.85, 43) -> (18.85, 64.2)
  line L13 (18.85, 64.2) -> (22.85, 64.2)
  line L14 (22.85, 64.2) -> (22.85, 43)
  dimension "d71" = 4
  dimension "d72" = 4
  dimension "d73" = 4
  dimension "d74" = 4
  constraint coincident L0.start L3.end
  constraint midpoint L0 L4.end
  constraint parallel L0 L5
  constraint horizontal L6
  constraint vertical L7
  constraint horizontal L8
  constraint vertical L9
  constraint parallel L4 L10
  constraint horizontal L11
  constraint vertical L12
  constraint horizontal L13
  constraint vertical L14
  measures "d71" distance of L4.end L5.end
  measures "d72" distance of L5.end L6.end
  measures "d73" distance of L4.end L10.end
  measures "d74" distance of L10.end L11.end
extrude "Extruir21" add sketch "Boceto21" along normal blind 4 contours L0 L2 L4 L11 L12 L13 L14 | L0 L2 L6 L7 L8 L9 bodies 1
sketch "Boceto22" plane through (41, 0, 0) normal (-1, 0, 0) x (0, 0, 1)
  line L0 (-70, 43) -> (16.3, 43)
  line L1 (16.3, 43) -> (16.3, 64.2)
  line L2 (16.3, 64.2) -> (-70, 64.2)
  line L3 (-70, 64.2) -> (-70, 43)
  line L4 (-30.85, 64.2) -> (-30.85, 43)
  line L5 (-34.85, 43) -> (-34.85, 64.2)
  line L6 (-34.85, 64.2) -> (-30.85, 64.2)
  line L7 (-18.85, 64.2) -> (-22.85, 64.2)
  line L8 (-22.85, 64.2) -> (-22.85, 43)
  line L9 (-18.85, 43) -> (-18.85, 64.2)
  line L10 (16.3, 43) -> (-26.85, 43)
  line L11 (-26.85, 43) -> (-30.85, 43)
  line L12 (-30.85, 43) -> (-34.85, 43)
extrude "Extruir22" add sketch "Boceto22" along normal blind 4 contours L0 L2 L4 L5 L6 L12 | L0 L2 L7 L8 L9 L10 bodies 1
sketch "Boceto23" plane through (0, 43, 0) normal (0, 1, 0) x (-1, 0, 0)
  line L0 (76, -30.85) -> (80, -30.85)
  line L1 (80, -30.85) -> (80, -22.85)
  line L2 (80, -22.85) -> (76, -22.85)
  line L3 (76, -22.85) -> (76, -18.85)
  line L4 (76, -18.85) -> (80, -18.85)
  line L5 (80, -18.85) -> (80, 16.3)
  line L6 (80, 16.3) -> (74, 16.3)
  line L7 (74, 16.3) -> (74, -70)
  line L8 (74, -70) -> (80, -70)
  line L9 (80, -70) -> (80, -34.85)
  line L10 (80, -34.85) -> (76, -34.85)
  line L11 (76, -34.85) -> (76, -30.85)
  line L12 (-41, 16.3) -> (80, 16.3)
  line L13 (80, 16.3) -> (80, -18.85)
  line L14 (80, -18.85) -> (76, -18.85)
  line L15 (76, -18.85) -> (76, -22.85)
  line L16 (76, -22.85) -> (80, -22.85)
  line L17 (80, -22.85) -> (80, -30.85)
  line L18 (80, -30.85) -> (76, -30.85)
  line L19 (76, -30.85) -> (76, -34.85)
  line L20 (76, -34.85) -> (80, -34.85)
  line L21 (80, -34.85) -> (80, -70)
  line L22 (80, -70) -> (-41, -70)
  line L23 (-41, -70) -> (-41, -34.85)
  line L24 (-41, -34.85) -> (-37, -34.85)
  line L25 (-37, -34.85) -> (-37, -30.85)
  line L26 (-37, -30.85) -> (-41, -30.85)
  line L27 (-41, -30.85) -> (-41, -22.85)
  line L28 (-41, -22.85) -> (-37, -22.85)
  line L29 (-37, -22.85) -> (-37, -18.85)
  line L30 (-37, -18.85) -> (-41, -18.85)
  line L31 (-41, -18.85) -> (-41, 16.3)
  line L32 (-44, -73) -> (83, -73)
  line L33 (83, -73) -> (83, 19.3)
  line L34 (83, 19.3) -> (-44, 19.3)
  line L35 (-44, 19.3) -> (-44, -73)
extrude "Extruir23" add sketch "Boceto23" along normal blind 3 separate body contours L0 L1 L2 L3 L4 L5 L6 L7 L8 L9 L10 L11 L12 L13 L14 L15 L16 L17 L18 L19 L20 L21 L22 | L7 L12 L22 L23 L24 L25 L26 L27 L28 L29 L30 L31 makes body 2
sketch "Boceto24" plane through (0, 46, 0) normal (0, 1, 0) x (-1, 0, 0)
  line L0 (-41, -18.85) -> (-37, -18.85)
  line L1 (-37, -18.85) -> (-37, -22.85)
  line L2 (-37, -22.85) -> (-41, -22.85)
  line L3 (-41, -22.85) -> (-41, -30.85)
  line L4 (-41, -30.85) -> (-37, -30.85)
  line L5 (-37, -30.85) -> (-37, -34.85)
  line L6 (-37, -34.85) -> (-41, -34.85)
  line L7 (-41, -34.85) -> (-41, -70)
  line L8 (-41, -70) -> (80, -70)
  line L9 (80, -70) -> (80, -34.85)
  line L10 (80, -34.85) -> (76, -34.85)
  line L11 (76, -34.85) -> (76, -30.85)
  line L12 (76, -30.85) -> (80, -30.85)
  line L13 (80, -30.85) -> (80, -22.85)
  line L14 (80, -22.85) -> (76, -22.85)
  line L15 (76, -22.85) -> (76, -18.85)
  line L16 (76, -18.85) -> (80, -18.85)
  line L17 (80, -18.85) -> (80, 16.3)
  line L18 (80, 16.3) -> (-41, 16.3)
  line L19 (-41, 16.3) -> (-41, -18.85)
  line L20 (31, 15.5) -> (51, 15.5)
  line L21 (51, -15.5) -> (31, -15.5)
  line L22 (-39, -41.65) -> (79, -41.65)
  line L23 (31, -15.5) -> (31, -16.5)
  line L24 (31, 16.5) -> (31, 15.5)
  circle A0 centre (75, -37.65) radius 3
  line L25 (79, -41.65) -> (79, 41.65)
  line L26 (79, 41.65) -> (-39, 41.65)
  line L27 (-39, 41.65) -> (-39, -41.65)
  line L28 (51, 15.5) -> (51, -15.5)
  line L29 (31, -16.5) -> (9, -16.5)
  line L30 (9, 16.5) -> (31, 16.5)
  line L31 (9, -16.5) -> (9, 16.5)
  circle A1 centre (-35, -37.65) radius 3
  line L32 (31, 5) -> (10, 5)
  line L33 (31, -5.5) -> (10, -5.5)
  line L34 (10, -5.5) -> (10, -15.5)
  line L35 (31, 5.5) -> (31, 15.5)
  line L36 (10, 5.5) -> (30, 5.5)
  line L37 (10, 15.5) -> (10, 5.5)
  line L38 (10, 5) -> (10, -5)
  line L39 (10, -5) -> (31, -5)
  line L40 (10, -15.5) -> (31, -15.5)
  line L41 (31, -15.5) -> (31, -5.5)
  line L42 (31, -5) -> (31, 5)
  line L43 (30, 5.5) -> (31, 5.5)
  circle A2 centre (75, 37.65) radius 3
  line L44 (31, 15.5) -> (10, 15.5)
  circle A3 centre (-35, 37.65) radius 3
  point P0 (20, 0)
sketch "Boceto25" plane through (0, 46, 0) normal (0, 1, 0) x (-1, 0, 0)
  line L0 (-41, -18.85) -> (-37, -18.85)
  line L1 (-37, -18.85) -> (-37, -22.85)
  line L2 (-37, -22.85) -> (-41, -22.85)
  line L3 (-41, -22.85) -> (-41, -30.85)
  line L4 (-41, -30.85) -> (-37, -30.85)
  line L5 (-37, -30.85) -> (-37, -34.85)
  line L6 (-37, -34.85) -> (-41, -34.85)
  line L7 (-41, -34.85) -> (-41, -70)
  line L8 (-41, -70) -> (80, -70)
  line L9 (80, -70) -> (80, -34.85)
  line L10 (80, -34.85) -> (76, -34.85)
  line L11 (76, -34.85) -> (76, -30.85)
  line L12 (76, -30.85) -> (80, -30.85)
  line L13 (80, -30.85) -> (80, -22.85)
  line L14 (80, -22.85) -> (76, -22.85)
  line L15 (76, -22.85) -> (76, -18.85)
  line L16 (76, -18.85) -> (80, -18.85)
  line L17 (80, -18.85) -> (80, 16.3)
  line L18 (80, 16.3) -> (-41, 16.3)
  line L19 (-41, 16.3) -> (-41, -18.85)
  line L20 (9, -10.35) -> (30, -10.35)
  line L21 (30, -10.35) -> (30, -43.35)
  line L22 (30, -43.35) -> (9, -43.35)
  line L23 (9, -43.35) -> (9, -10.35)
  line L24 (9, -10.35) -> (30, -43.35) construction
  line L25 (30, -10.35) -> (9, -43.35) construction
  line L26 (80, -70) -> (-41, 16.3) construction
  line L27 (80, 16.3) -> (-41, -70) construction
  line L28 (30, -43.35) -> (30, -43.35)
  line L29 (30, -43.35) -> (30, -42.35)
  line L30 (30, -42.35) -> (30, -42.35)
  line L31 (30, -42.35) -> (30, -43.35)
  line L32 (30, -42.35) -> (10, -42.35)
  line L33 (10, -42.35) -> (10, -11.35)
  line L34 (10, -11.35) -> (30, -11.35)
  line L35 (10, -42.35) -> (10, -32.35)
  line L36 (10, -32.35) -> (30, -32.35)
  line L37 (10, -32.35) -> (10, -31.35)
  line L38 (10, -31.35) -> (30, -31.35)
  line L39 (9, -31.35) -> (9, -21.35)
  line L40 (9, -21.35) -> (30, -21.35)
  line L41 (10, -21.35) -> (10, -20.35)
  line L42 (10, -20.35) -> (30, -20.35)
  point P0 (19.5, -26.85)
  dimension "d81" = 33
  dimension "d82" = 21
  dimension "d83" = 1
  dimension "d84" = 31
  dimension "d85" = 10
  dimension "d86" = 1
  dimension "d87" = 10
  dimension "d88" = 1
  constraint horizontal L20
  constraint perpendicular L20 L21
  constraint parallel L20 L22
  constraint parallel L21 L23
  constraint coincident L24 P0
  constraint coincident L25 P0
  constraint coincident L8.end L9.start
  constraint coincident L18.end L19.start
  constraint coincident L17.end L18.start
  constraint coincident L7.end L8.start
  constraint coincident P0 L27
  constraint coincident P0 L26
  constraint vertical L29
  constraint vertical L31
  constraint perpendicular L21 L32
  constraint perpendicular L32 L33
  constraint coincident L21 L34.end
  constraint perpendicular L21 L34
  constraint perpendicular L32 L35
  constraint coincident L21 L36.end
  constraint perpendicular L21 L36
  constraint perpendicular L36 L37
  constraint coincident L21 L38.end
  constraint perpendicular L21 L38
  constraint coincident L23 L39.start
  constraint perpendicular L38 L39
  constraint coincident L21 L40.end
  constraint perpendicular L21 L40
  constraint coincident L40 L41.start
  constraint coincident L33 L41.start
  constraint perpendicular L40 L41
  constraint coincident L21 L42.end
  constraint perpendicular L21 L42
  measures "d81" distance of L20.start L22.end
  measures "d82" distance of L21.end L22.end
  measures "d83" distance of L21.end L29.end
  measures "d84" distance of L32.end L33.end
  measures "d85" distance of L32.end L35.end
  measures "d86" distance of L35.end L37.end
  measures "d87" distance of L39.start L39.end
  measures "d88" distance of L41.start L41.end
extrude "Extruir24" add sketch "Boceto25" along normal blind 20 contours L20 L21 L23 L33 L34 L40 L41 | L21 L22 L23 L29 L31 L32 L33 L35 L37 L39 L40 | L21 L33 L40 L41 L42 | L21 L33 L36 L37 L38 bodies 2
sketch "Boceto26" plane through (-19.5, 46, -26.85) normal (0, 1, 0) x (-1, 0, 0)
  line L0 (10.5, 16.5) -> (10.5, -16.5)
  line L1 (10.5, -15.5) -> (-9.5, -15.5)
  line L2 (-9.5, 15.5) -> (10.5, 15.5)
  line L3 (10.5, -15.5) -> (40.5, -15.5)
  line L4 (40.5, -15.5) -> (40.5, 15.5)
  line L5 (40.5, 15.5) -> (10.5, 15.5)
  line L6 (10.5, 15.5) -> (10.5, -15.5)
  point P0 (10.5, 15.5)
  dimension "d91" = 30
  constraint horizontal L3
  constraint vertical L4
  constraint horizontal L5
  constraint vertical L6
  constraint coincident L1.start L3.start
  constraint coincident P0 L2.end
  measures "d91" distance of L1.start L3.end
extrude "Extruir25" cut sketch "Boceto26" against normal blind 5 bodies 2
sketch "Boceto27" plane through (0, 66, 0) normal (0, 1, 0) x (-1, 0, 0)
  line L0 (10, -11.35) -> (30, -11.35)
  line L1 (30, -11.35) -> (30, -10.35)
  line L2 (30, -10.35) -> (9, -10.35)
  line L3 (9, -10.35) -> (9, -43.35)
  line L4 (9, -43.35) -> (30, -43.35)
  line L5 (30, -43.35) -> (30, -42.35)
  line L6 (30, -42.35) -> (10, -42.35)
  line L7 (10, -42.35) -> (10, -32.35)
  line L8 (10, -32.35) -> (30, -32.35)
  line L9 (30, -32.35) -> (30, -31.35)
  line L10 (30, -31.35) -> (10, -31.35)
  line L11 (10, -31.35) -> (10, -21.35)
  line L12 (10, -21.35) -> (30, -21.35)
  line L13 (30, -21.35) -> (30, -20.35)
  line L14 (30, -20.35) -> (10, -20.35)
  line L15 (10, -20.35) -> (10, -11.35)
  line L16 (-4.7, -11.65) -> (43.7, -11.65)
  line L17 (43.7, -11.65) -> (43.7, -42.05)
  line L18 (43.7, -42.05) -> (-4.7, -42.05)
  line L19 (-4.7, -42.05) -> (-4.7, -11.65)
  line L20 (-4.7, -11.65) -> (43.7, -42.05) construction
  line L21 (43.7, -11.65) -> (-4.7, -42.05) construction
  point P0 (19.5, -26.85)
  point P1 (19.5, -26.85)
  dimension "d94" = 30.4
  dimension "d95" = 48.4
  constraint horizontal L16
  constraint perpendicular L16 L17
  constraint parallel L16 L18
  constraint parallel L17 L19
  constraint coincident L20 P1
  constraint coincident L21 P1
  constraint coincident P1 P0
  measures "d94" distance of L16.start L18.end
  measures "d95" distance of L17.end L18.end
extrude "Extruir26" add sketch "Boceto27" along normal blind 2 contours L7 L8 L9 L10 L11 L12 L13 L14 L15 L16 L17 L18 | L3 L7 L8 L9 L10 L11 L12 L13 L14 L15 L16 L18 | L3 L16 L18 L19 bodies 2